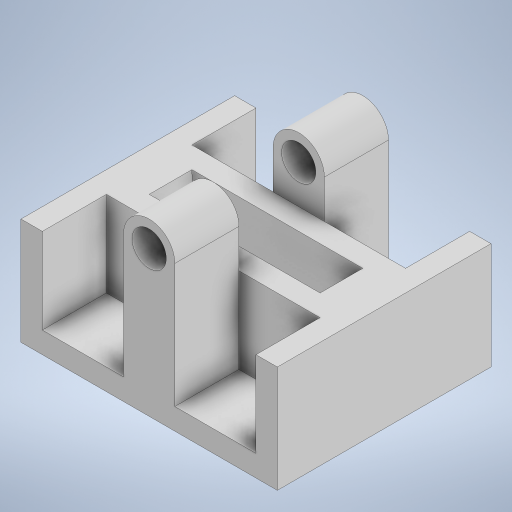
# Autodesk Inventor part: khurramf_01_Base
Saved by Autodesk Inventor 2024 (Build 280153000, 153)
## iProperties
Created: 2024-01-30
Part Number: khurramf_01_Base
Material: Generic
Document SubType Name: Modeling
Designer: furqa
Density: 1 g/cm^3
Appearance: Default
Author: furqa
Autodesk Inventor part; units mm, degrees
ref_plane "YZ Plane" through (0, 0, 0) normal (1, 0, 0) x (0, 1, 0)
ref_plane "XZ Plane" through (0, 0, 0) normal (0, 1, 0) x (-1, 0, 0)
sketch "Sketch2" plane through (0, 0, 0) normal (0, 0, 1) x (1, 0, 0)
  line L0 (30, -13.3137) -> (-30, -13.3137)
  line L1 (-30, -13.3137) -> (-30, 11.6863)
  line L2 (30, 11.6863) -> (30, -13.3137)
  line L3 (-25, 11.6863) -> (-30, 11.6863)
  line L4 (-6, 11.6863) -> (-6, 20.6863)
  line L5 (6, 20.6863) -> (6, 11.6863)
  arc A0 (6, 20.6863) -> (-6, 20.6863) centre (0, 20.6863) ccw
  circle A1 centre (0, 20.6863) radius 4
  line L6 (-30, 11.6863) -> (-6, 11.6863)
  line L7 (6, 11.6863) -> (30, 11.6863)
  point P0 (0, 0)
  dimension "d0" = 60
  dimension "d9" = 25
  dimension "d12" = 8
  dimension "d13" = 12
  dimension "d14" = 9
  constraints: 16 end point, 4 parallel, 2 centre point, 2 perpendicular, 2 point on circle, 1 coincident, 1 horizontal, 1 point on line
  measures "d0" distance of L1.end L2.start
  measures "d9" distance of L0.end L1.end
  measures "d12" diameter of A1
  measures "d13" diameter of A0
  measures "d14" distance of L5.start L5.end
extrude "Extrusion1" add sketch "Sketch2" along normal blind 25
sketch "Sketch3" plane through (0, 0, 0) normal (0, 0, -1) x (-1, 0, 0)
  line L0 (-25, 11.6863) -> (-6, 11.6863)
  line L1 (-6, 11.6863) -> (-6, -8.3137)
  line L2 (-6, -8.3137) -> (-25, -8.3137)
  line L3 (-25, -8.3137) -> (-25, 11.6863)
  line L4 (25, 11.6863) -> (6, 11.6863)
  line L5 (6, 11.6863) -> (6, -8.3137)
  line L6 (6, -8.3137) -> (25, -8.3137)
  line L7 (25, -8.3137) -> (25, 11.6863)
  line L8 (30, -13.3137) -> (-30, -13.3137) projected
  line L9 (-30, -13.3137) -> (-30, 11.6863) projected
  line L10 (30, 11.6863) -> (30, -13.3137) projected
  point P0 (0, 0)
  point P1 (-30, -0.8137)
  dimension "d17" = 5
  dimension "d18" = 5
  dimension "d19" = 5
  dimension "d20" = 5
  constraints: 16 end point, 4 parallel, 2 horizontal, 2 perpendicular, 1 midpoint
  measures "d17" distance between parallel lines of L8 L2
  measures "d18" distance from line of point (-30, -0.814) L3
  measures "d19" distance between parallel lines of L8 L6
  measures "d20" distance between parallel lines of L10 L7
extrude "Extrusion2" cut sketch "Sketch3" against normal blind 15
sketch "Sketch4" plane through (0, 0, 25) normal (0, 0, 1) x (1, 0, 0)
  line L0 (-6, 11.6863) -> (6, 11.6863)
  line L1 (6, 11.6863) -> (6, 20.6863)
  line L2 (6, 26.6863) -> (0, 26.6863)
  line L3 (-6, 20.6863) -> (-6, 11.6863)
  arc A0 (6, 20.6863) -> (-6, 20.6863) centre (0, 20.6863) ccw
  circle A1 centre (0, 20.6863) radius 4
  point P0 (0, 0)
  dimension "d23" = 15
  constraints: 8 end point, 3 point on circle, 2 centre point, 2 parallel, 1 coincident, 1 horizontal, 1 perpendicular
  measures "d23" distance of L2.start L0.end
extrude "Extrusion3" cut sketch "Sketch4" against normal blind 10
sketch "Sketch5" plane through (-30, 11.6863, 25) normal (0, 1, 0) x (1, 0, 0)
  line L0 (0, 0) -> (60, 0) projected
  line L1 (30, 0) -> (50, 0)
  line L2 (50, 0) -> (50, 5)
  line L3 (50, 5) -> (30, 5)
  line L4 (30, 5) -> (30, 0)
  point P0 (30, 25)
  dimension "d27" = 20
  dimension "d28" = 5
  constraints: 8 end point, 2 parallel, 1 horizontal, 1 midpoint, 1 perpendicular
  measures "d27" distance of L3.end L2.end
  measures "d28" distance of L1.end L2.end
revolve "Revolution1" cut sketch "Sketch5" angle 360 about axis through (0, 11.6863, 20) along (0, 0, 1)
ref_plane "Work Plane1" through (0, 0, 25) normal (0, 0, 1) x (1, 0, 0)
mirror "Mirror1" about plane through (0, 0, 25) normal (0, 0, 1)
body "Solid1"
